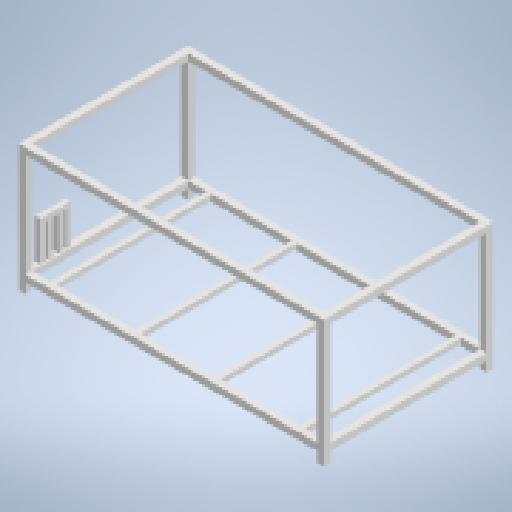
# Autodesk Inventor part: BangTai
Saved by Autodesk Inventor 2023 (Build 270158000, 158)
## iProperties
Created: 2025-03-24
Part Number: BangTai
Material: Generic
Document SubType Name: Modeling
Designer: huyqu
Density: 1 g/cm^3
Appearance: Default
Author: huyqu
Autodesk Inventor part; units mm, degrees
ref_plane "YZ Plane" through (0, 0, 0) normal (1, 0, 0) x (0, 1, 0)
ref_plane "XZ Plane" through (0, 0, 0) normal (0, 1, 0) x (-1, 0, 0)
ref_plane "XY Plane" through (0, 0, 0) normal (0, 0, 1) x (1, 0, 0)
sketch "Sketch1" plane through (0, 0, 0) normal (0, 0, 1) x (1, 0, 0)
  line L0 (0, 0) -> (1800, 0)
  line L1 (0, 0) -> (0, -40)
  line L2 (0, -40) -> (1800, -40)
  line L3 (1800, -40) -> (1800, 0)
  dimension "d0" = 1800
  dimension "d1" = 40
  constraints: 8 end point, 1 horizontal, 1 parallel, 1 perpendicular, 1 vertical
  measures "d0" distance of L0.start L0.end
  measures "d1" distance of L0.start L1.end
extrude "Extrusion1" add sketch "Sketch1" along normal blind 40
sketch "Sketch2" plane through (0, 0, 40) normal (0, 0, 1) x (1, 0, 0)
  line L0 (0, 0) -> (0, -40) projected
  line L1 (1800, 0) -> (0, 0) projected
  line L2 (0, 0) -> (40, 0)
  line L3 (0, -40) -> (1800, -40) projected
  line L4 (40, -40) -> (0, -40)
  line L5 (0, -40) -> (0, 0)
  line L6 (40, 0) -> (40, -40)
  line L7 (1800, -40) -> (1800, 0) projected
  line L8 (1800, 0) -> (1760, 0)
  line L9 (1760, -40) -> (1800, -40)
  line L10 (1760, 0) -> (1760, -40)
  line L11 (1800, 0) -> (1800, -40)
  dimension "d5" = 40
  dimension "d6" = 40
  constraints: 16 end point, 4 collinear, 4 point on line, 1 perpendicular, 1 vertical
  measures "d5" distance between parallel lines of L6 L0
  measures "d6" distance between parallel lines of L7 L10
extrude "Extrusion2" add sketch "Sketch2" along normal blind 960 contours L1 L6 L3 L0 | L1 L7 L3 L10
sketch "Sketch4" plane through (1760, -40, 40) normal (-1, 0, 0) x (0, 0, 1)
  line L0 (960, 40) -> (960, 0) projected
  line L1 (960, 40) -> (920, 40)
  line L2 (0, 40) -> (960, 40) projected
  line L3 (0, 0) -> (960, 0) projected
  line L4 (920, 0) -> (920, 40)
  line L5 (920, 0) -> (960, 0)
  line L6 (960, 0) -> (960, 40)
  point P0 (-40, 40)
  dimension "d9" = 40
  constraints: 8 end point, 2 perpendicular, 2 point on line, 1 horizontal
  measures "d9" distance between parallel lines of L0 L4
extrude "Extrusion3" add sketch "Sketch4" along normal up to surface (1720 mm away)
sketch "Sketch5" plane through (0, -40, 0) normal (0, -1, 0) x (1, 0, 0)
  line L0 (40, 40) -> (40, 960) projected
  line L1 (40, 960) -> (40, 1000)
  line L2 (1800, 1000) -> (0, 1000) projected
  line L3 (0, 1000) -> (0, 960)
  line L4 (0, 0) -> (0, 1000) projected
  line L5 (40, 960) -> (0, 960)
  line L6 (0, 1000) -> (40, 1000)
  line L7 (1760, 40) -> (1760, 960) projected
  line L8 (1760, 960) -> (1800, 960)
  line L9 (1800, 0) -> (1800, 1000) projected
  line L10 (1760, 960) -> (1760, 1000)
  line L11 (1760, 1000) -> (1800, 1000)
  line L12 (1800, 1000) -> (1800, 960)
  line L13 (1760, 40) -> (40, 40) projected
  line L14 (1760, 40) -> (1800, 40)
  line L15 (1800, 40) -> (1800, 0)
  line L16 (1800, 0) -> (1760, 0)
  line L17 (1800, 0) -> (0, 0) projected
  line L18 (1760, 0) -> (1760, 40)
  line L19 (0, 40) -> (40, 40)
  line L20 (40, 0) -> (40, 40)
  line L21 (0, 40) -> (0, 0)
  line L22 (40, 0) -> (0, 0)
  constraints: 32 end point, 15 point on line, 7 perpendicular, 2 parallel, 1 vertical
extrude "Extrusion4" add sketch "Sketch5" along normal blind 710 contours L20 L17 L4 L19 | L5 L3 L2 L1 | L14 L9 L16 L18 | L10 L2 L9 L8
sketch "Sketch6" plane through (1760, -40, 0) normal (-1, 0, 0) x (0, 0, 1)
  line L0 (0, 40) -> (0, -710) projected
  line L1 (0, -610) -> (40, -610)
  line L2 (40, 0) -> (40, -710) projected
  line L3 (0, -610) -> (0, -650)
  line L4 (0, -650) -> (40, -650)
  line L5 (40, -650) -> (40, -610)
  line L6 (0, 0) -> (40, 0) projected
  line L7 (960, 0) -> (960, -710) projected
  line L8 (960, -610) -> (1000, -610)
  line L9 (1000, 0) -> (1000, -710) projected
  line L10 (960, -650) -> (1000, -650)
  line L11 (1000, -650) -> (1000, -610)
  line L12 (960, -610) -> (960, -650)
  dimension "d14" = 40
  dimension "d15" = 650
  constraints: 16 end point, 4 point on line, 3 horizontal, 3 perpendicular, 1 parallel, 1 vertical
  measures "d14" distance between parallel lines of L4 L1
  measures "d15" distance between parallel lines of L4 L6
extrude "Extrusion5" add sketch "Sketch6" along normal up to surface (1720 mm away) contours L1 L2 L4 L0 | L8 L9 L10 L7
sketch "Sketch7" plane through (0, -750, 40) normal (0, 0, 1) x (1, 0, 0)
  line L0 (40, 710) -> (40, 100) projected
  line L1 (40, 100) -> (0, 100)
  line L2 (0, 100) -> (0, 60)
  line L3 (40, 60) -> (40, 0) projected
  line L4 (0, 60) -> (40, 60)
  line L5 (40, 60) -> (40, 100)
  line L6 (1760, 60) -> (1760, 0) projected
  line L7 (1760, 60) -> (1800, 60)
  line L8 (1800, 710) -> (1800, 0) projected
  line L9 (1760, 710) -> (1760, 100) projected
  line L10 (1800, 100) -> (1760, 100)
  line L11 (1760, 100) -> (1760, 60)
  line L12 (0, 100) -> (0, 60)
  line L13 (0, 710) -> (0, 0) projected
  line L14 (1800, 100) -> (1800, 60)
  line L15 (0, 100) -> (0, 60)
  point P0 (0, 750)
  constraints: 20 end point, 4 point on line, 3 perpendicular, 2 collinear, 2 horizontal, 1 parallel, 1 vertical
extrude "Extrusion6" add sketch "Sketch7" along normal up to surface (920 mm away)
sketch "Sketch8" plane through (0, 0, 0) normal (-1, 0, 0) x (0, 0, 1)
  line L0 (40, -650) -> (960, -650) projected
  line L1 (902, -650) -> (902, -420)
  line L2 (902, -420) -> (722, -420)
  line L3 (722, -420) -> (722, -650)
  line L4 (960, -40) -> (960, -650) projected
  line L5 (722, -450) -> (902, -450)
  line L6 (722, -650) -> (902, -650)
  line L7 (764.1942, -450) -> (764.1942, -650)
  line L8 (794.1942, -450) -> (794.1942, -650)
  line L9 (826.1942, -450) -> (826.1942, -650)
  line L10 (856.1942, -450) -> (856.1942, -650)
  line L11 (872.1942, -450) -> (872.1942, -650)
  line L12 (748.1942, -450) -> (748.1942, -650)
  point P0 (0, 0)
  dimension "d20" = 230
  dimension "d21" = 58
  dimension "d22" = 180
  dimension "d23" = 30
  dimension "d24" = 30
  dimension "d25" = 30
  dimension "d26" = 32
  dimension "d27" = 16
  dimension "d28" = 16
  constraints: 22 end point, 16 point on line, 9 perpendicular, 1 horizontal, 1 vertical
  measures "d20" distance of L1.start L1.end
  measures "d21" distance between parallel lines of L4 L1
  measures "d22" distance of L1.end L2.end
  measures "d23" distance between parallel lines of L5 L2
  measures "d24" distance between parallel lines of L8 L7
  measures "d25" distance between parallel lines of L10 L9
  measures "d26" distance between parallel lines of L9 L8
  measures "d27" distance between parallel lines of L11 L10
  measures "d28" distance between parallel lines of L7 L12
extrude "Extrusion7" add sketch "Sketch8" against normal blind 30 contours L3 L5 L12 L0 | L3 L2 L1 L5 | L7 L5 L8 L0 | L9 L5 L10 L0 | L1 L0 L11 L5
sketch "Sketch9" plane through (1760, -690, 960) normal (0, 0, -1) x (-1, 0, 0)
  line L0 (0, 40) -> (1720, 40) projected
  line L1 (110, 40) -> (140, 40)
  line L2 (140, 40) -> (140, 10)
  line L3 (140, 10) -> (110, 10)
  line L4 (110, 10) -> (110, 40)
  line L5 (610, 40) -> (640, 40)
  line L6 (640, 40) -> (640, 10)
  line L7 (640, 10) -> (610, 10)
  line L8 (610, 10) -> (610, 40)
  line L9 (1080, 40) -> (1110, 40)
  line L10 (1110, 40) -> (1110, 10)
  line L11 (1110, 10) -> (1080, 10)
  line L12 (1080, 10) -> (1080, 40)
  line L13 (1580, 40) -> (1610, 40)
  line L14 (1610, 40) -> (1610, 10)
  line L15 (1610, 10) -> (1580, 10)
  line L16 (1580, 10) -> (1580, 40)
  line L17 (-40, -60) -> (-40, 690) projected
  line L18 (1760, 690) -> (1760, -60) projected
  point P0 (1610, 40)
  point P1 (1580, 40)
  point P2 (640, 40)
  point P3 (610, 40)
  dimension "d31" = 30
  dimension "d32" = 30
  dimension "d33" = 30
  dimension "d34" = 30
  dimension "d35" = 30
  dimension "d36" = 30
  dimension "d37" = 30
  dimension "d38" = 30
  dimension "d39" = 150
  dimension "d40" = 150
  dimension "d41" = 470
  dimension "d42" = 470
  constraints: 32 end point, 8 parallel, 4 horizontal, 4 perpendicular, 1 point on line
  measures "d31" distance of L3.end L1.start
  measures "d32" distance between parallel lines of L2 L4
  measures "d33" distance of L7.end L5.start
  measures "d34" distance between parallel lines of L6 L8
  measures "d35" distance of L11.end L9.start
  measures "d36" distance between parallel lines of L10 L12
  measures "d37" distance of L15.end L13.start
  measures "d38" distance between parallel lines of L14 L16
  measures "d39" distance between parallel lines of L17 L4
  measures "d40" distance between parallel lines of L18 L14
  measures "d41" distance between parallel lines of L16 L10
  measures "d42" distance between parallel lines of L8 L2
extrude "Extrusion8" add sketch "Sketch9" along normal up to surface (920 mm away)
sketch "Sketch24" plane through (0, -750, 0) normal (0, -1, 0) x (1, 0, 0)
  circle A0 centre (20, 20) radius 6
  line L0 (40, 40) -> (0, 40) projected
  line L1 (0, 40) -> (0, 0) projected
  point P0 (0, 20)
  dimension "d95" = 20
  dimension "d96" = 20
  dimension "d97" = 12
  constraints: 1 centre point, 1 midpoint
  measures "d95" distance from line of A0.centre L0
  measures "d96" distance of point (0, 20) A0.centre
  measures "d97" diameter of A0
sketch "Sketch25" plane through (0, -750, 0) normal (0, -1, 0) x (1, 0, 0)
  circle A0 centre (20, 980) radius 6
  line L0 (40, 1000) -> (0, 1000) projected
  line L1 (0, 1000) -> (0, 960) projected
  circle A1 centre (1780, 980) radius 6
  circle A2 centre (1780, 20) radius 6
  line L2 (1760, 0) -> (1800, 0) projected
  line L3 (1800, 0) -> (1800, 40) projected
  point P0 (0, 0)
  dimension "d98" = 20
  dimension "d99" = 20
  dimension "d100" = 12
  dimension "d101" = 20
  dimension "d102" = 20
  dimension "d103" = 12
  constraints: 3 centre point
  measures "d98" distance from line of A0.centre L0
  measures "d99" distance from line of A0.centre L1
  measures "d100" diameter of A0
  measures "d101" distance from line of L2 A2.centre
  measures "d102" distance from line of L3 A2.centre
  measures "d103" diameter of A2
hole "Hole1" at (20, -750, 20) direction (0, 1, 0) diameter 12 depth 20 tip angle 118
hole "Hole2" at (20, -750, 980) at (1780, -750, 980) at (1780, -750, 20) direction (0, 1, 0) diameter 12 depth 20 tip angle 118
body "Solid1"
